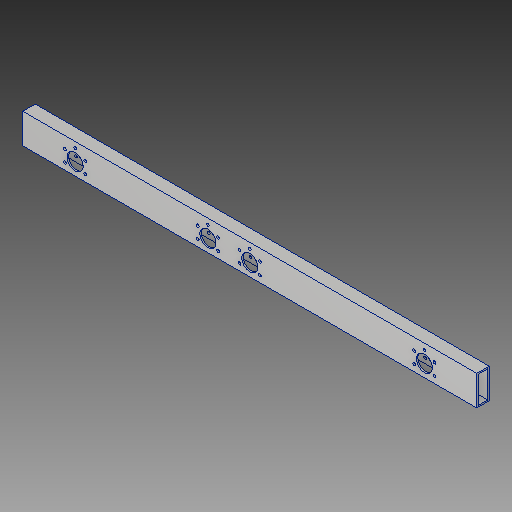
# Autodesk Inventor part: Main Extrusion
Saved by Autodesk Inventor 2019.4 (Build 234330000, 330)
## iProperties
Created: 2020-01-05
Part Number: Main Extrusion
Material: Aluminum 6061
Document SubType Name: Modeling
Designer: Mark
Mass: 1104.81 g
Surface Area: 2782.26 cm^2
Volume: 409.187 cm^3
Density: 2.7 g/cm^3
Appearance: Aluminum - Flat
Author: Mark
Autodesk Inventor part; units mm, degrees
ref_plane "YZ Plane" through (0, 0, 0) normal (1, 0, 0) x (0, 1, 0)
ref_plane "XZ Plane" through (0, 0, 0) normal (0, 1, 0) x (-1, 0, 0)
ref_plane "XY Plane" through (0, 0, 0) normal (0, 0, 1) x (1, 0, 0)
sketch "Sketch1" plane through (0, 0, 0) normal (1, 0, 0) x (0, 1, 0)
  line L0 (-30, 12.5) -> (30, 12.5)
  line L1 (30, 12.5) -> (30, -12.5)
  line L2 (30, -12.5) -> (-30, -12.5)
  line L3 (-30, -12.5) -> (-30, 12.5)
  line L4 (-30, 12.5) -> (30, -12.5) construction
  line L5 (30, 12.5) -> (-30, -12.5) construction
  line L6 (-27, 9.5) -> (27, 9.5)
  line L7 (27, 9.5) -> (27, -9.5)
  line L8 (27, -9.5) -> (-27, -9.5)
  line L9 (-27, -9.5) -> (-27, 9.5)
  line L10 (-27, 9.5) -> (27, -9.5) construction
  line L11 (27, 9.5) -> (-27, -9.5) construction
  point P0 (0, 0)
  dimension "d0" = 60
  dimension "d1" = 25
  dimension "d2" = 54
  dimension "d3" = 19
  constraints: 24 end point, 4 midpoint, 4 parallel, 2 horizontal, 2 perpendicular
  measures "d0" distance of L1.end L2.end
  measures "d1" distance of L0.end L1.end
  measures "d2" distance of L7.end L8.end
  measures "d3" distance of L6.end L7.end
extrude "Extrusion1" add sketch "Sketch1" along normal blind 910
sketch "Sketch2" plane through (0, -30, 12.5) normal (0, 0, 1) x (1, 0, 0)
  circle A0 centre (455, 25) radius 16
  circle A1 centre (105, 25) radius 16
  circle A2 centre (805, 25) radius 16
  line L0 (0, 0) -> (0, 60) projected
  line L1 (0, 0) -> (910, 0) projected
  circle A3 centre (371, 25) radius 16
  circle A4 centre (455, 25) radius 23.5 construction
  line L2 (455, 25) -> (455, 1.5) construction
  line L3 (455, 25) -> (478.5, 25) construction
  circle A5 centre (455, 1.5) radius 2.75
  circle A6 centre (475.3516, 13.25) radius 2.75
  circle A7 centre (475.3516, 36.75) radius 2.75
  circle A8 centre (455, 48.5) radius 2.75
  circle A9 centre (434.6484, 36.75) radius 2.75
  circle A10 centre (434.6484, 13.25) radius 2.75
  circle A11 centre (371, 25) radius 23.5 construction
  line L4 (371, 25) -> (371, 1.5) construction
  line L5 (371, 25) -> (394.5, 25) construction
  circle A12 centre (391.3516, 13.25) radius 2.75
  circle A13 centre (391.3516, 36.75) radius 2.75
  circle A14 centre (371, 48.5) radius 2.75
  circle A15 centre (350.6484, 36.75) radius 2.75
  circle A16 centre (350.6484, 13.25) radius 2.75
  circle A17 centre (371, 1.5) radius 2.75
  circle A18 centre (105, 25) radius 23.5 construction
  line L6 (105, 25) -> (105, 1.5) construction
  line L7 (105, 25) -> (128.5, 25) construction
  circle A19 centre (105, 1.5) radius 2.75
  circle A20 centre (125.3516, 13.25) radius 2.75
  circle A21 centre (125.3516, 36.75) radius 2.75
  circle A22 centre (105, 48.5) radius 2.75
  circle A23 centre (84.6484, 36.75) radius 2.75
  circle A24 centre (84.6484, 13.25) radius 2.75
  circle A25 centre (805, 25) radius 23.5 construction
  line L8 (805, 25) -> (805, 1.5) construction
  circle A26 centre (805, 1.5) radius 2.75
  circle A27 centre (825.3516, 13.25) radius 2.75
  circle A28 centre (825.3516, 36.75) radius 2.75
  circle A29 centre (805, 48.5) radius 2.75
  circle A30 centre (784.6484, 36.75) radius 2.75
  circle A31 centre (784.6484, 13.25) radius 2.75
  point P0 (0, 30)
  dimension "d22" = 47
  dimension "d36" = 47
  dimension "d43" = 47
  dimension "d6" = 32
  dimension "d7" = 32
  dimension "d8" = 32
  dimension "d9" = 455
  dimension "d10" = 25
  dimension "d13" = 25
  dimension "d14" = 25
  dimension "d18" = 32
  dimension "d19" = 25
  dimension "d20" = 84
  dimension "d21" = 266
  dimension "d23" = 90
  dimension "d24" = 5.5
  dimension "d27" = 360
  dimension "d29" = 47
  dimension "d30" = 90
  dimension "d31" = 5.5
  dimension "d34" = 360
  dimension "d37" = 90
  dimension "d38" = 5.5
  dimension "d41" = 360
  dimension "d44" = 350
  dimension "d45" = 5.5
  dimension "d48" = 360
  constraints: 29 centre point, 14 end point, 8 coincident, 3 horizontal, 3 perpendicular, 3 vertical alignment, 2 point on circle, 1 vertical, 58 other
  measures "d6" diameter of A0
  measures "d7" diameter of A1
  measures "d8" diameter of A2
  measures "d9" distance from line of L0 A0.centre
  measures "d10" distance from line of L1 A0.centre
  measures "d13" distance from line of L1 A1.centre
  measures "d14" distance from line of L1 A2.centre
  measures "d18" diameter of A3
  measures "d19" distance from line of L1 A3.centre
  measures "d20" distance of A0.centre A3.centre
  measures "d21" distance of A3.centre A1.centre
  measures "d23" angle of L2 L3
  measures "d24" diameter of A5
  measures "d29" diameter of A11
  measures "d30" angle of L4 L5
  measures "d31" diameter of A12
  measures "d37" angle of L6 L7
  measures "d38" diameter of A19
  measures "d44" distance of A0.centre A2.centre
  measures "d45" diameter of A26
extrude "Extrusion2" cut sketch "Sketch2" against normal blind 30 contours A0 | A1 | A2 | A3 | A6 | A7 | A8 | A9 | A10 | A12 | A13 | A14 | A15 | A16 | A20 | A21 | A22 | A23 | A24 | A27 | A28 | A29 | A30 | A31
equation "\"d13\" = d10"
equation "\"d14\" = d10"
equation "\"d19\" = d10"
equation "\"d21\" = d11 - d20"
equation "\"d11\" = 350"
body "Solid1"
